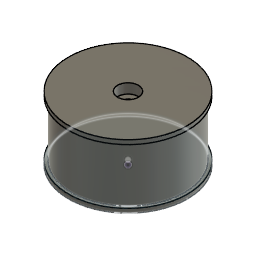
OTIS wheel for silicon band (Autodesk Fusion 360 design; units mm, degrees)
part number: 2026-08-18-21-24-11-877
Autodesk Fusion 360 part; units mm, degrees
note: some values were not read from the file. Chosen so that the rebuilt part matches the saved one: which bodies a step acts on.
sketch "Sketch1" plane through (0, 0, 0) normal (0, 1, 0) x (1, 0, 0)
  circle A0 centre (0, 0) radius 14
  dimension "d1" = 28
  constraint coincident A0.centre origin
  measures "d1" diameter of A0
extrude "Extrude1" add sketch "Sketch1" along normal blind 15 makes body 1
shell "Shell1" thickness 1 removed faces 1 at (13.9304, 10, 1.3939) on bodies 1 makes body 2 at (4.6394, 0, -2.5701)
sketch "Sketch2" plane through (0, 1, 0) normal (0, 1, 0) x (-1, 0, 0)
  circle A0 centre (0, 0) radius 14
  circle A1 centre (0, 0) radius 13.35
  dimension "d5" = 26.7
  constraint concentric A0 A1
  measures "d5" diameter of A1
extrude "Extrude2" add sketch "Sketch2" along normal blind 13 contours A1 bodies 1 2
sketch "Sketch3" plane through (0, 15, 0) normal (0, 1, 0) x (-1, 0, 0)
  circle A0 centre (0, 0) radius 14
  circle A1 centre (0, 0) radius 2.45
  dimension "d8" = 4.9
  constraint coincident A0.centre A1.centre
  measures "d8" diameter of A1
extrude "Extrude3" cut sketch "Sketch3" against normal blind 2.3 contours A1 bodies 1
sketch "Sketch4" plane through (0, 12.7, 0) normal (0, 1, 0) x (-1, 0, 0)
  circle A0 centre (0, 0) radius 2.45
  circle A1 centre (0, 0) radius 1.05
  dimension "d11" = 2.1
  constraint coincident A0.centre A1.centre
  measures "d11" diameter of A1
extrude "Extrude4" cut sketch "Sketch4" against normal blind 39.33 contours A1 bodies 1
